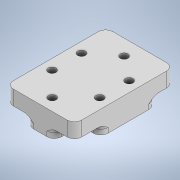
# Autodesk Inventor part: Cartridge Internal - Top Cover 2
Saved by Autodesk Inventor 2021 (Build 250183000, 183)
## iProperties
Created: 2020-05-07
Part Number: Cartridge Internal - Top Cover 2
Material: Generic
Document SubType Name: Modeling
Designer: jgray
Density: 1 g/cm^3
Appearance: Default
Author: jgray
Autodesk Inventor part; units mm, degrees
ref_plane "YZ Plane" through (0, 0, 0) normal (1, 0, 0) x (0, 1, 0)
ref_plane "XZ Plane" through (0, 0, 0) normal (0, 1, 0) x (-1, 0, 0)
ref_plane "XY Plane" through (0, 0, 0) normal (0, 0, 1) x (1, 0, 0)
sketch "Sketch1" plane through (0, 0, 0) normal (0, 1, 0) x (-1, 0, 0)
  line L0 (13.9, -32.7368) -> (-13.9, -32.7368)
  line L1 (13.9, 35.0132) -> (13.9, -32.7368)
  line L2 (-13.9, 35.0132) -> (13.9, 35.0132)
  line L3 (-13.9, -32.7368) -> (-13.9, 35.0132)
  circle A0 centre (9.4, -30.5) radius 1.7
  circle A1 centre (-9.4, -15) radius 1.7
  circle A2 centre (9.4, 15) radius 1.7
  circle A3 centre (-9.4, 15) radius 1.7
  circle A4 centre (-9.4, 30.5) radius 1.7
  circle A5 centre (9.4, 30.5) radius 1.7
  circle A6 centre (9.4, -15) radius 1.7
  circle A7 centre (-9.4, -30.5) radius 1.7
  line L4 (0, 45.3153) -> (0, -54.1069) construction
  line L5 (-30.6732, 0) -> (30.6732, 0) construction
  line L6 (0, 65.0497) -> (0, -74.1413)
  line L7 (13.9, 35.0132) -> (-13.9, 35.0132)
  line L8 (-13.9, 35.0132) -> (-13.9, -18.5)
  line L9 (-13.9, -18.5) -> (13.9, -18.5)
  line L10 (13.9, -18.5) -> (13.9, 35.0132)
  line L11 (-13.9, 22) -> (13.9, 22)
  point P0 (0, 0)
  point P1 (0, 0)
  point P2 (0, 0)
  point P3 (0, 17.15)
  point P4 (-9.7, 7)
  point P5 (9.7, 7)
  point P6 (-10.4, -6)
  point P7 (10.4, -6)
  point P8 (0, -12.15)
  point P9 (13.9, 22)
  dimension "d1" = 7
  dimension "d2" = 7
  dimension "d3" = 4.2
  dimension "d4" = 4.2
  dimension "d5" = 3.5
  dimension "d6" = 3.5
  dimension "d7" = 12.15
  dimension "d10" = 3.5
  dimension "d11" = 15
  dimension "d58" = 22
  dimension "d59" = 13
  dimension "d60" = 13
  dimension "d61" = 17.15
  constraints: 24 end point, 8 centre point, 7 point on line, 2 horizontal, 2 midpoint, 2 parallel, 2 perpendicular, 1 vertical
  measures "d1" distance from line of point (9.7, 7) L5
  measures "d2" distance from line of point (-9.7, 7) L5
  measures "d3" distance from line of L3 point (-9.7, 7)
  measures "d4" distance from line of L1 point (9.7, 7)
  measures "d5" distance from line of L1 point (10.4, -6)
  measures "d6" distance from line of L3 point (-10.4, -6)
  measures "d7" distance from line of point (0, -12.15) L5
  measures "d10" distance from line of L9 A1.centre
  measures "d11" distance from line of A1.centre L5
  measures "d58" distance between parallel lines of L11 L5
  measures "d59" vertical distance of point (10.4, -6) point (9.7, 7)
  measures "d60" vertical distance of point (-10.4, -6) point (-9.7, 7)
  measures "d61" distance from line of point (0, 17.15) L5
extrude "Extrusion1" add sketch "Sketch1" along normal blind 10 contours L9 L6 L11 L1 | L9 L3 L11 L6 | A1 | A2 | A3 | A6
sketch "Sketch2" plane through (0, 0, 0) normal (0, -1, 0) x (1, 0, 0)
  line L0 (13.9, -32.7368) -> (-13.9, -32.7368)
  line L1 (13.9, 35.0132) -> (13.9, -32.7368)
  line L2 (-13.9, 35.0132) -> (13.9, 35.0132)
  line L3 (-13.9, -32.7368) -> (-13.9, 35.0132)
  circle A0 centre (9.4, -30.5) radius 1.7
  circle A1 centre (-9.4, -15) radius 1.7
  circle A2 centre (9.4, 15) radius 1.7
  circle A3 centre (-9.4, 15) radius 1.7
  circle A4 centre (-9.4, 30.5) radius 1.7
  circle A5 centre (9.4, 30.5) radius 1.7
  circle A6 centre (9.4, -15) radius 1.7
  circle A7 centre (-9.4, -30.5) radius 1.7
  line L4 (0, 45.3153) -> (0, -54.1069) construction
  line L5 (-30.6732, 0) -> (30.6732, 0) construction
  line L6 (0, 65.0497) -> (0, -74.1413)
  line L7 (13.9, 35.0132) -> (-13.9, 35.0132)
  line L8 (-13.9, 35.0132) -> (-13.9, -18.5)
  line L9 (-13.9, -18.5) -> (13.9, -18.5)
  line L10 (13.9, -18.5) -> (13.9, 35.0132)
  circle A8 centre (0, 17.15) radius 1.6
  circle A9 centre (9.7, 7.5) radius 1.6
  circle A10 centre (9.7, -4.5) radius 1.6
  circle A11 centre (-9.7, -4.5) radius 1.6
  circle A12 centre (0, -12.15) radius 1.6
  circle A13 centre (-9.7, 7.5) radius 1.6
  point P0 (0, 0)
  point P1 (0, 0)
  point P2 (0, 0)
  point P3 (0, 0)
  dimension "d15" = 7.5
  dimension "d16" = 7.5
  dimension "d17" = 4.2
  dimension "d18" = 4.2
  dimension "d19" = 4.2
  dimension "d20" = 4.2
  dimension "d21" = 12.15
  dimension "d24" = 3.5
  dimension "d25" = 15
  dimension "d26" = 3.2
  dimension "d27" = 3.2
  dimension "d28" = 3.2
  dimension "d29" = 3.2
  dimension "d30" = 3.2
  dimension "d31" = 3.2
  dimension "d62" = 12
  dimension "d63" = 12
  dimension "d64" = 17.15
  constraints: 22 end point, 14 centre point, 6 coincident, 5 point on line, 2 horizontal, 2 midpoint, 2 parallel, 1 perpendicular, 1 vertical
  measures "d15" distance from line of point (9.7, 7.5) L5
  measures "d16" distance from line of point (-9.7, 7.5) L5
  measures "d17" distance from line of L3 point (-9.7, 7.5)
  measures "d18" distance from line of L1 point (9.7, 7.5)
  measures "d19" distance from line of L1 point (9.7, -4.5)
  measures "d20" distance from line of L3 point (-9.7, -4.5)
  measures "d21" distance from line of point (0, -12.15) L5
  measures "d24" distance from line of L9 A1.centre
  measures "d25" distance from line of A1.centre L5
  measures "d26" diameter of A8
  measures "d27" diameter of A9
  measures "d28" diameter of A10
  measures "d29" diameter of A11
  measures "d30" diameter of A12
  measures "d31" diameter of A13
  measures "d62" distance of A9.centre point (9.7, -4.5)
  measures "d63" distance of A11.centre A13.centre
  measures "d64" distance from line of A8.centre L5
extrude "Extrusion2" cut sketch "Sketch2" against normal through all contours A12 L6 | L6 A12 | A8 L6 | L6 A8 | A9 | A10 | A11 | A13
sketch "Sketch3" plane through (0, 0, 0) normal (0, -1, 0) x (1, 0, 0)
  line L0 (13.9, -32.7368) -> (-13.9, -32.7368)
  line L1 (13.9, 22) -> (13.9, -32.7368)
  line L2 (-13.9, -32.7368) -> (-13.9, 22)
  circle A0 centre (9.4, -30.5) radius 1.7
  circle A1 centre (-9.4, -15) radius 1.7
  circle A2 centre (9.4, 15) radius 1.7
  circle A3 centre (-9.4, 15) radius 1.7
  circle A4 centre (9.4, -15) radius 1.7
  circle A5 centre (-9.4, -30.5) radius 1.7
  line L3 (0, 45.3153) -> (0, -54.1069) construction
  line L4 (-30.6732, 0) -> (30.6732, 0) construction
  line L5 (0, 65.1997) -> (0, -73.9913)
  line L6 (-13.9, 22) -> (-13.9, -18.5)
  line L7 (-13.9, -18.5) -> (13.9, -18.5)
  arc A6 (5.7, 15) -> (9.4, 11.3) centre (9.4, 15) ccw
  arc A7 (-9.4, 11.3) -> (-5.7, 15) centre (-9.4, 15) ccw
  line L8 (13.9, 22) -> (13.9, -18.5) projected
  line L9 (9.4, 11.3) -> (13.9, 11.3)
  line L10 (-13.9, -18.5) -> (-13.9, 22) projected
  line L11 (-9.4, 11.3) -> (-13.9, 11.3)
  line L12 (-5.7, -15) -> (-5.7, -18.5)
  line L13 (-9.4, -11.3) -> (-13.9, -11.3)
  line L14 (9.4, -11.3) -> (13.9, -11.3)
  line L15 (5.7, -15) -> (5.7, -18.7)
  arc A8 (9.4, -11.3) -> (5.7, -15) centre (9.4, -15) ccw
  arc A9 (-5.7, -15) -> (-9.4, -11.3) centre (-9.4, -15) ccw
  circle A10 centre (-9.7, 7.5) radius 1.6 projected
  circle A11 centre (0, -12.15) radius 1.6 projected
  circle A12 centre (9.7, 7.5) radius 1.6 projected
  circle A13 centre (9.7, -4.5) radius 1.6 projected
  circle A14 centre (-9.7, -4.5) radius 1.6 projected
  circle A15 centre (0, 17.15) radius 1.6 projected
  line L16 (-13.9, -18.5) -> (-13.9, 22) projected
  line L17 (13.9, -18.5) -> (-13.9, -18.5) projected
  line L18 (13.9, 22) -> (13.9, -18.5) projected
  line L19 (-13.9, 22) -> (13.9, 22) projected
  line L20 (13.9, -18.5) -> (13.9, 22)
  line L21 (5.7, 15) -> (5.7, 22)
  line L22 (-5.7, 15) -> (-5.7, 22)
  line L23 (-13.9, 22) -> (13.9, 22) projected
  point P0 (0, 0)
  point P1 (0, 0)
  point P2 (0, 0)
  point P3 (0, 0)
  point P4 (0, -12)
  point P5 (13.9, -18.5)
  point P6 (5.7, -18.5)
  point P7 (13.9, -18.5)
  dimension "d41" = 12
  dimension "d44" = 3.5
  dimension "d45" = 15
  dimension "d47" = 7.4
  dimension "d50" = 7.4
  constraints: 35 end point, 17 point on line, 10 centre point, 8 point on circle, 3 perpendicular, 3 tangent, 2 midpoint, 2 parallel, 2 vertical, 1 horizontal
  measures "d41" distance from line of point (0, -12) L4
  measures "d44" distance from line of L7 A1.centre
  measures "d45" distance from line of A1.centre L4
  measures "d47" diameter of A6
  measures "d50" diameter of A7
extrude "Extrusion3" cut sketch "Sketch3" against normal blind 4 contours L7 L15 A8 L14 L1 | L2 L13 A9 L12 L7 | L9 A6 L21 L19 L1 | L2 L19 L22 A7 L11 | A1 | A2 | A3 | A4
fillet "Fillet2" radius 3 8 edges at (13.9, 2, 11.3) (-13.9, 2, 11.3) (13.9, 2, -11.3) (5.7, 2, -18.5) (-13.9, 2, -11.3) (-5.7, 2, -18.5) (5.7, 2, 22) (-5.7, 2, 22)
fillet "Fillet3" radius 2 16 edges at (10.15, 4, 11.3) (13.0213, 4, 10.4213) (6.7837, 4, 12.3837) (-10.15, 4, 11.3) (-6.7837, 4, 12.3837) (-13.0213, 4, 10.4213) (6.7837, 4, -12.3837) (10.15, 4, -11.3) (13.0213, 4, -10.4213) (4.8213, 4, -17.6213) (5.7, 4, -15.25) (-5.7, 4, -15.25) (-4.8213, 4, -17.6213) (-10.15, 4, -11.3) (-13.0213, 4, -10.4213) (-6.7837, 4, -12.3837)
fillet "Fillet4" radius 3 4 edges at (-13.9, 7, -18.5) (13.9, 7, -18.5) (13.9, 7, 22) (-13.9, 7, 22)
equation "\"d2\" = d1"
equation "\"d60\" = d59"
equation "\"d15\" = d16"
equation "\"d63\" = d62"
body "Solid1"
